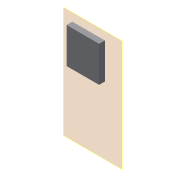
# Autodesk Inventor part: 30_cellSTORM_UC2_motorized_xystage_coupler_fibermount
Saved by Autodesk Inventor 2022 (Build 260153000, 153)
## iProperties
Created: 2021-10-28
Part Number: 30_cellSTORM_UC2_motorized_xystage_coupler_fibermount
Material: Generic
Document SubType Name: Modeling
Designer: diederichbenedict
Density: 1 g/cm^3
Appearance: Default
Author: diederichbenedict
Autodesk Inventor part; units mm, degrees
ref_plane "YZ Plane" through (0, 0, 0) normal (1, 0, 0) x (0, 1, 0)
ref_plane "XZ Plane" through (0, 0, 0) normal (0, 1, 0) x (-1, 0, 0)
ref_plane "XY Plane" through (0, 0, 0) normal (0, 0, 1) x (1, 0, 0)
ref_plane "Work Plane1" through (0, 0, 0) normal (0, 0, 1) x (1, 0, 0)
sketch "Sketch1" plane through (0, 0, 0) normal (0, 0, 1) x (1, 0, 0)
  circle A0 centre (5.5332, 19.4257) radius 2.45 construction
  circle A1 centre (-14.4668, 30.9727) radius 2.45 construction
  circle A2 centre (5.5332, 42.5198) radius 2.45 construction
  line L0 (12.5332, 12.4257) -> (-21.4668, 12.4257)
  line L1 (-21.4668, 12.4257) -> (-21.4668, 49.5198)
  line L2 (-21.4668, 49.5198) -> (12.5332, 49.5198)
  line L3 (12.5332, 49.5198) -> (12.5332, 12.4257)
  circle A3 centre (5.5332, 19.4257) radius 2.45
  circle A4 centre (-14.4668, 30.9727) radius 2.45
  circle A5 centre (5.5332, 42.5198) radius 2.45
  point P0 (0, 0)
  dimension "d0" = 7
  dimension "d1" = 7
  dimension "d2" = 7
  dimension "d3" = 7
  dimension "d4" = 4.9
  dimension "d5" = 4.9
  dimension "d6" = 4.9
  constraints: 8 end point, 3 centre point, 3 coincident, 2 parallel, 1 horizontal, 1 perpendicular
  measures "d0" distance from line of L0 A0.centre
  measures "d1" distance from line of L2 A2.centre
  measures "d2" distance from line of A1.centre L1
  measures "d3" distance from line of A0.centre L3
  measures "d4" diameter of A3
  measures "d5" diameter of A4
  measures "d6" diameter of A5
extrude "Extrusion1" add sketch "Sketch1" along normal blind 4
sketch "Sketch2" plane through (0, 0, 4) normal (0, 0, 1) x (1, 0, 0)
  line L0 (12.5332, 49.5198) -> (-21.4668, 49.5198) projected
  line L1 (-21.4668, 49.5198) -> (-21.4668, 12.4257) projected
  line L2 (-21.4668, 12.4257) -> (12.5332, 12.4257) projected
  line L3 (12.5332, 12.4257) -> (12.5332, 49.5198) projected
  circle A0 centre (5.5332, 42.5198) radius 2.45 projected
  circle A1 centre (-14.4668, 30.9727) radius 2.45 projected
  circle A2 centre (5.5332, 19.4257) radius 2.45 projected
  point P0 (0, 0)
extrude "Extrusion2" add sketch "Sketch2" along normal blind 2 contours L3 L2 L1 L0 | A0 | A1 | A2
sketch "Sketch3" plane through (-21.4668, 12.4257, 0) normal (-1, 0, 0) x (0, 0, 1)
  line L0 (0, 37.094) -> (0, 0) projected
  line L1 (0, 0) -> (6, 0) projected
  line L2 (6, 37.094) -> (6, 0) projected
  line L3 (0, 37.094) -> (6, 37.094) projected
  line L4 (0, 37.094) -> (6, 37.094) projected
  line L5 (6, 37.094) -> (15, 37.094)
  line L6 (15, 37.094) -> (15, 0)
  line L7 (15, 0) -> (6, 0)
  line L8 (6, 0) -> (6, 37.094)
  circle A0 centre (10.5, 18.8104) radius 1.5
  point P0 (0, -12.4257)
  dimension "d11" = 9
  dimension "d12" = 3
  constraints: 8 end point, 2 parallel, 1 centre point, 1 horizontal, 1 perpendicular
  measures "d11" distance of L6.end L7.end
  measures "d12" diameter of A0
extrude "Extrusion3" add sketch "Sketch3" against normal blind 10 contours L5 L6 L7 L2
sketch "Sketch4" plane through (-21.4668, 12.4257, 0) normal (-1, 0, 0) x (0, 0, 1)
  line L0 (7.55, 24.4104) -> (13.45, 24.4104) projected
  line L1 (13.45, 14.3104) -> (7.55, 14.3104) projected
  line L2 (13.45, 24.4104) -> (7.55, 24.4104)
  line L3 (7.55, 24.4104) -> (7.55, 14.3104)
  line L4 (7.55, 14.3104) -> (13.45, 14.3104)
  line L5 (13.45, 14.3104) -> (13.45, 24.4104)
  line L6 (13.65, 24.6104) -> (7.35, 24.6104)
  line L7 (7.35, 24.6104) -> (7.35, 14.1104)
  line L8 (7.35, 14.1104) -> (13.65, 14.1104)
  line L9 (13.65, 14.1104) -> (13.65, 24.6104)
  point P0 (0, -12.4257)
  dimension "d15" = 0.2
  constraints: 16 end point, 4 parallel, 2 perpendicular, 1 horizontal, 3 other
  measures "d15" distance between parallel lines of L5 L9
extrude "Extrusion4" cut sketch "Sketch4" against normal blind 10 contours L0 L5 L1 L3 | L9 L8 L7 L6
sketch "Sketch5" plane through (-21.4668, 49.5198, 0) normal (0, 1, 0) x (1, 0, 0)
  line L0 (9.45, -4) -> (4.55, -4) projected
  line L1 (34, 0) -> (0, 0) projected
  line L2 (0, 0) -> (0, -15) projected
  line L3 (0, -15) -> (10, -15) projected
  line L4 (10, -6) -> (10, -15) projected
  line L5 (34, -6) -> (10, -6) projected
  line L6 (34, 0) -> (34, -6) projected
  circle A0 centre (5, -10.5) radius 1.4
  point P0 (21.4668, 0)
  point P1 (4.9, -8.2)
  dimension "d18" = 2.8
  constraints: 1 centre point, 1 other
  measures "d18" diameter of A0
extrude "Extrusion5" cut sketch "Sketch5" against normal through all contours A0
sketch "Sketch6" plane through (0, 0, 6) normal (0, 0, 1) x (1, 0, 0)
  line L0 (-11.4668, 49.5198) -> (-11.4668, 12.4257) projected
  line L1 (-11.4668, 12.4257) -> (12.5332, 12.4257) projected
  line L2 (12.5332, 12.4257) -> (12.5332, 49.5198) projected
  line L3 (12.5332, 49.5198) -> (-11.4668, 49.5198) projected
  circle A0 centre (-14.4668, 30.9727) radius 2.45 projected
  circle A1 centre (5.5332, 42.5198) radius 2.45 projected
  circle A2 centre (5.5332, 33.4727) radius 1.4
  circle A3 centre (5.5332, 28.4727) radius 1.4
  point P0 (0, 0)
  dimension "d21" = 2.8
  dimension "d22" = 2.8
  dimension "d23" = 2.5
  dimension "d24" = 2.5
  constraints: 2 centre point
  measures "d21" diameter of A2
  measures "d22" diameter of A3
  measures "d23" vertical distance of A2.centre A0.centre
  measures "d24" vertical distance of A0.centre A3.centre
extrude "Extrusion6" cut sketch "Sketch6" along normal through all both and the other way through all contours A2 | A3
equation "\"d5\" = d4"
equation "\"d6\" = d4"
body "Solid1"
